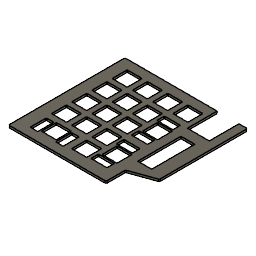
numpad (Autodesk Fusion 360 archive; units mm, degrees)
design "middle"
part number: 2026-06-12-14-33-51-478
Autodesk Fusion 360 part; units mm, degrees
sketch "Sketch2" plane through (0, 0, 0) normal (0, 0, 1) x (1, 0, 0)
  line L0 (-33.9143, 32.5199) -> (-20.9143, 32.5199)
  line L1 (-33.9143, 18.5199) -> (-20.9143, 18.5199)
  line L2 (-34.4143, 32.0199) -> (-34.4143, 19.0199)
  line L3 (-20.4143, 32.0199) -> (-20.4143, 19.0199)
  arc A0 (-33.9143, 32.5199) -> (-34.4143, 32.0199) centre (-33.9143, 32.0199) ccw
  arc A1 (-20.4143, 32.0199) -> (-20.9143, 32.5199) centre (-20.9143, 32.0199) ccw
  arc A2 (-34.4143, 19.0199) -> (-33.9143, 18.5199) centre (-33.9143, 19.0199) ccw
  arc A3 (-20.9143, 18.5199) -> (-20.4143, 19.0199) centre (-20.9143, 19.0199) ccw
  line L4 (-14.8643, 32.5199) -> (-1.8643, 32.5199)
  line L5 (-14.8643, 18.5199) -> (-1.8643, 18.5199)
  line L6 (-15.3643, 32.0199) -> (-15.3643, 19.0199)
  line L7 (-1.3643, 32.0199) -> (-1.3643, 19.0199)
  arc A4 (-14.8643, 32.5199) -> (-15.3643, 32.0199) centre (-14.8643, 32.0199) ccw
  arc A5 (-1.3643, 32.0199) -> (-1.8643, 32.5199) centre (-1.8643, 32.0199) ccw
  arc A6 (-15.3643, 19.0199) -> (-14.8643, 18.5199) centre (-14.8643, 19.0199) ccw
  arc A7 (-1.8643, 18.5199) -> (-1.3643, 19.0199) centre (-1.8643, 19.0199) ccw
  line L8 (4.1857, 32.5199) -> (17.1857, 32.5199)
  line L9 (4.1857, 18.5199) -> (17.1857, 18.5199)
  line L10 (3.6857, 32.0199) -> (3.6857, 19.0199)
  line L11 (17.6857, 32.0199) -> (17.6857, 19.0199)
  arc A8 (4.1857, 32.5199) -> (3.6857, 32.0199) centre (4.1857, 32.0199) ccw
  arc A9 (17.6857, 32.0199) -> (17.1857, 32.5199) centre (17.1857, 32.0199) ccw
  arc A10 (3.6857, 19.0199) -> (4.1857, 18.5199) centre (4.1857, 19.0199) ccw
  arc A11 (17.1857, 18.5199) -> (17.6857, 19.0199) centre (17.1857, 19.0199) ccw
  line L12 (23.2357, 32.5199) -> (36.2357, 32.5199)
  line L13 (23.2357, 18.5199) -> (36.2357, 18.5199)
  line L14 (22.7357, 32.0199) -> (22.7357, 19.0199)
  line L15 (36.7357, 32.0199) -> (36.7357, 19.0199)
  arc A12 (23.2357, 32.5199) -> (22.7357, 32.0199) centre (23.2357, 32.0199) ccw
  arc A13 (36.7357, 32.0199) -> (36.2357, 32.5199) centre (36.2357, 32.0199) ccw
  arc A14 (22.7357, 19.0199) -> (23.2357, 18.5199) centre (23.2357, 19.0199) ccw
  arc A15 (36.2357, 18.5199) -> (36.7357, 19.0199) centre (36.2357, 19.0199) ccw
  line L16 (-33.9143, 13.4699) -> (-20.9143, 13.4699)
  line L17 (-33.9143, -0.5301) -> (-20.9143, -0.5301)
  line L18 (-34.4143, 12.9699) -> (-34.4143, -0.0301)
  line L19 (-20.4143, 12.9699) -> (-20.4143, -0.0301)
  arc A16 (-33.9143, 13.4699) -> (-34.4143, 12.9699) centre (-33.9143, 12.9699) ccw
  arc A17 (-20.4143, 12.9699) -> (-20.9143, 13.4699) centre (-20.9143, 12.9699) ccw
  arc A18 (-34.4143, -0.0301) -> (-33.9143, -0.5301) centre (-33.9143, -0.0301) ccw
  arc A19 (-20.9143, -0.5301) -> (-20.4143, -0.0301) centre (-20.9143, -0.0301) ccw
  line L20 (-14.8643, 13.4699) -> (-1.8643, 13.4699)
  line L21 (-14.8643, -0.5301) -> (-1.8643, -0.5301)
  line L22 (-15.3643, 12.9699) -> (-15.3643, -0.0301)
  line L23 (-1.3643, 12.9699) -> (-1.3643, -0.0301)
  arc A20 (-14.8643, 13.4699) -> (-15.3643, 12.9699) centre (-14.8643, 12.9699) ccw
  arc A21 (-1.3643, 12.9699) -> (-1.8643, 13.4699) centre (-1.8643, 12.9699) ccw
  arc A22 (-15.3643, -0.0301) -> (-14.8643, -0.5301) centre (-14.8643, -0.0301) ccw
  arc A23 (-1.8643, -0.5301) -> (-1.3643, -0.0301) centre (-1.8643, -0.0301) ccw
  line L24 (4.1857, 13.4699) -> (17.1857, 13.4699)
  line L25 (4.1857, -0.5301) -> (17.1857, -0.5301)
  line L26 (3.6857, 12.9699) -> (3.6857, -0.0301)
  line L27 (17.6857, 12.9699) -> (17.6857, -0.0301)
  arc A24 (4.1857, 13.4699) -> (3.6857, 12.9699) centre (4.1857, 12.9699) ccw
  arc A25 (17.6857, 12.9699) -> (17.1857, 13.4699) centre (17.1857, 12.9699) ccw
  arc A26 (3.6857, -0.0301) -> (4.1857, -0.5301) centre (4.1857, -0.0301) ccw
  arc A27 (17.1857, -0.5301) -> (17.6857, -0.0301) centre (17.1857, -0.0301) ccw
  line L28 (36.7357, 3.4449) -> (36.7357, -9.5551)
  line L29 (22.7357, 3.4449) -> (22.7357, -9.5551)
  line L30 (36.2357, 3.9449) -> (23.2357, 3.9449)
  line L31 (36.2357, -10.0551) -> (23.2357, -10.0551)
  arc A28 (36.7357, 3.4449) -> (36.2357, 3.9449) centre (36.2357, 3.4449) ccw
  arc A29 (36.2357, -10.0551) -> (36.7357, -9.5551) centre (36.2357, -9.5551) ccw
  arc A30 (23.2357, 3.9449) -> (22.7357, 3.4449) centre (23.2357, 3.4449) ccw
  arc A31 (22.7357, -9.5551) -> (23.2357, -10.0551) centre (23.2357, -9.5551) ccw
  line L32 (35.7357, 11.8829) -> (35.7357, 5.8829)
  line L33 (20.7357, 11.8829) -> (20.7357, 5.8829)
  line L34 (35.2357, 12.3829) -> (21.2357, 12.3829)
  line L35 (35.2357, 5.3829) -> (21.2357, 5.3829)
  arc A32 (35.7357, 11.8829) -> (35.2357, 12.3829) centre (35.2357, 11.8829) ccw
  arc A33 (35.2357, 5.3829) -> (35.7357, 5.8829) centre (35.2357, 5.8829) ccw
  arc A34 (21.2357, 12.3829) -> (20.7357, 11.8829) centre (21.2357, 11.8829) ccw
  arc A35 (20.7357, 5.8829) -> (21.2357, 5.3829) centre (21.2357, 5.8829) ccw
  line L36 (35.7357, -11.9931) -> (35.7357, -17.9931)
  line L37 (20.7357, -11.9931) -> (20.7357, -17.9931)
  line L38 (35.2357, -11.4931) -> (21.2357, -11.4931)
  line L39 (35.2357, -18.4931) -> (21.2357, -18.4931)
  arc A36 (35.7357, -11.9931) -> (35.2357, -11.4931) centre (35.2357, -11.9931) ccw
  arc A37 (35.2357, -18.4931) -> (35.7357, -17.9931) centre (35.2357, -17.9931) ccw
  arc A38 (21.2357, -11.4931) -> (20.7357, -11.9931) centre (21.2357, -11.9931) ccw
  arc A39 (20.7357, -17.9931) -> (21.2357, -18.4931) centre (21.2357, -17.9931) ccw
  line L40 (-33.9143, -5.5801) -> (-20.9143, -5.5801)
  line L41 (-33.9143, -19.5801) -> (-20.9143, -19.5801)
  line L42 (-34.4143, -6.0801) -> (-34.4143, -19.0801)
  line L43 (-20.4143, -6.0801) -> (-20.4143, -19.0801)
  arc A40 (-33.9143, -5.5801) -> (-34.4143, -6.0801) centre (-33.9143, -6.0801) ccw
  arc A41 (-20.4143, -6.0801) -> (-20.9143, -5.5801) centre (-20.9143, -6.0801) ccw
  arc A42 (-34.4143, -19.0801) -> (-33.9143, -19.5801) centre (-33.9143, -19.0801) ccw
  arc A43 (-20.9143, -19.5801) -> (-20.4143, -19.0801) centre (-20.9143, -19.0801) ccw
  line L44 (-14.8643, -5.5801) -> (-1.8643, -5.5801)
  line L45 (-14.8643, -19.5801) -> (-1.8643, -19.5801)
  line L46 (-15.3643, -6.0801) -> (-15.3643, -19.0801)
  line L47 (-1.3643, -6.0801) -> (-1.3643, -19.0801)
  arc A44 (-14.8643, -5.5801) -> (-15.3643, -6.0801) centre (-14.8643, -6.0801) ccw
  arc A45 (-1.3643, -6.0801) -> (-1.8643, -5.5801) centre (-1.8643, -6.0801) ccw
  arc A46 (-15.3643, -19.0801) -> (-14.8643, -19.5801) centre (-14.8643, -19.0801) ccw
  arc A47 (-1.8643, -19.5801) -> (-1.3643, -19.0801) centre (-1.8643, -19.0801) ccw
  line L48 (4.1857, -5.5801) -> (17.1857, -5.5801)
  line L49 (4.1857, -19.5801) -> (17.1857, -19.5801)
  line L50 (3.6857, -6.0801) -> (3.6857, -19.0801)
  line L51 (17.6857, -6.0801) -> (17.6857, -19.0801)
  arc A48 (4.1857, -5.5801) -> (3.6857, -6.0801) centre (4.1857, -6.0801) ccw
  arc A49 (17.6857, -6.0801) -> (17.1857, -5.5801) centre (17.1857, -6.0801) ccw
  arc A50 (3.6857, -19.0801) -> (4.1857, -19.5801) centre (4.1857, -19.0801) ccw
  arc A51 (17.1857, -19.5801) -> (17.6857, -19.0801) centre (17.1857, -19.0801) ccw
  line L52 (-33.9143, -24.6301) -> (-20.9143, -24.6301)
  line L53 (-33.9143, -38.6301) -> (-20.9143, -38.6301)
  line L54 (-34.4143, -25.1301) -> (-34.4143, -38.1301)
  line L55 (-20.4143, -25.1301) -> (-20.4143, -38.1301)
  arc A52 (-33.9143, -24.6301) -> (-34.4143, -25.1301) centre (-33.9143, -25.1301) ccw
  arc A53 (-20.4143, -25.1301) -> (-20.9143, -24.6301) centre (-20.9143, -25.1301) ccw
  arc A54 (-34.4143, -38.1301) -> (-33.9143, -38.6301) centre (-33.9143, -38.1301) ccw
  arc A55 (-20.9143, -38.6301) -> (-20.4143, -38.1301) centre (-20.9143, -38.1301) ccw
  line L56 (-14.8643, -24.6301) -> (-1.8643, -24.6301)
  line L57 (-14.8643, -38.6301) -> (-1.8643, -38.6301)
  line L58 (-15.3643, -25.1301) -> (-15.3643, -38.1301)
  line L59 (-1.3643, -25.1301) -> (-1.3643, -38.1301)
  arc A56 (-14.8643, -24.6301) -> (-15.3643, -25.1301) centre (-14.8643, -25.1301) ccw
  arc A57 (-1.3643, -25.1301) -> (-1.8643, -24.6301) centre (-1.8643, -25.1301) ccw
  arc A58 (-15.3643, -38.1301) -> (-14.8643, -38.6301) centre (-14.8643, -38.1301) ccw
  arc A59 (-1.8643, -38.6301) -> (-1.3643, -38.1301) centre (-1.8643, -38.1301) ccw
  line L60 (4.1857, -24.6301) -> (17.1857, -24.6301)
  line L61 (4.1857, -38.6301) -> (17.1857, -38.6301)
  line L62 (3.6857, -25.1301) -> (3.6857, -38.1301)
  line L63 (17.6857, -25.1301) -> (17.6857, -38.1301)
  arc A60 (4.1857, -24.6301) -> (3.6857, -25.1301) centre (4.1857, -25.1301) ccw
  arc A61 (17.6857, -25.1301) -> (17.1857, -24.6301) centre (17.1857, -25.1301) ccw
  arc A62 (3.6857, -38.1301) -> (4.1857, -38.6301) centre (4.1857, -38.1301) ccw
  arc A63 (17.1857, -38.6301) -> (17.6857, -38.1301) centre (17.1857, -38.1301) ccw
  line L64 (36.7357, -34.6551) -> (36.7357, -47.6551)
  line L65 (22.7357, -34.6551) -> (22.7357, -47.6551)
  line L66 (36.2357, -34.1551) -> (23.2357, -34.1551)
  line L67 (36.2357, -48.1551) -> (23.2357, -48.1551)
  arc A64 (36.7357, -34.6551) -> (36.2357, -34.1551) centre (36.2357, -34.6551) ccw
  arc A65 (36.2357, -48.1551) -> (36.7357, -47.6551) centre (36.2357, -47.6551) ccw
  arc A66 (23.2357, -34.1551) -> (22.7357, -34.6551) centre (23.2357, -34.6551) ccw
  arc A67 (22.7357, -47.6551) -> (23.2357, -48.1551) centre (23.2357, -47.6551) ccw
  line L68 (35.7357, -26.2171) -> (35.7357, -32.2171)
  line L69 (20.7357, -26.2171) -> (20.7357, -32.2171)
  line L70 (35.2357, -25.7171) -> (21.2357, -25.7171)
  line L71 (35.2357, -32.7171) -> (21.2357, -32.7171)
  arc A68 (35.7357, -26.2171) -> (35.2357, -25.7171) centre (35.2357, -26.2171) ccw
  arc A69 (35.2357, -32.7171) -> (35.7357, -32.2171) centre (35.2357, -32.2171) ccw
  arc A70 (21.2357, -25.7171) -> (20.7357, -26.2171) centre (21.2357, -26.2171) ccw
  arc A71 (20.7357, -32.2171) -> (21.2357, -32.7171) centre (21.2357, -32.2171) ccw
  line L72 (35.7357, -50.0931) -> (35.7357, -56.0931)
  line L73 (20.7357, -50.0931) -> (20.7357, -56.0931)
  line L74 (35.2357, -49.5931) -> (21.2357, -49.5931)
  line L75 (35.2357, -56.5931) -> (21.2357, -56.5931)
  arc A72 (35.7357, -50.0931) -> (35.2357, -49.5931) centre (35.2357, -50.0931) ccw
  arc A73 (35.2357, -56.5931) -> (35.7357, -56.0931) centre (35.2357, -56.0931) ccw
  arc A74 (21.2357, -49.5931) -> (20.7357, -50.0931) centre (21.2357, -50.0931) ccw
  arc A75 (20.7357, -56.0931) -> (21.2357, -56.5931) centre (21.2357, -56.0931) ccw
  line L76 (-24.3893, -43.6801) -> (-11.3893, -43.6801)
  line L77 (-24.3893, -57.6801) -> (-11.3893, -57.6801)
  line L78 (-24.8893, -44.1801) -> (-24.8893, -57.1801)
  line L79 (-10.8893, -44.1801) -> (-10.8893, -57.1801)
  arc A76 (-24.3893, -43.6801) -> (-24.8893, -44.1801) centre (-24.3893, -44.1801) ccw
  arc A77 (-10.8893, -44.1801) -> (-11.3893, -43.6801) centre (-11.3893, -44.1801) ccw
  arc A78 (-24.8893, -57.1801) -> (-24.3893, -57.6801) centre (-24.3893, -57.1801) ccw
  arc A79 (-11.3893, -57.6801) -> (-10.8893, -57.1801) centre (-11.3893, -57.1801) ccw
  line L80 (-32.8273, -44.6801) -> (-26.8273, -44.6801)
  line L81 (-32.8273, -59.6801) -> (-26.8273, -59.6801)
  line L82 (-33.3273, -45.1801) -> (-33.3273, -59.1801)
  line L83 (-26.3273, -45.1801) -> (-26.3273, -59.1801)
  arc A80 (-32.8273, -44.6801) -> (-33.3273, -45.1801) centre (-32.8273, -45.1801) ccw
  arc A81 (-26.3273, -45.1801) -> (-26.8273, -44.6801) centre (-26.8273, -45.1801) ccw
  arc A82 (-33.3273, -59.1801) -> (-32.8273, -59.6801) centre (-32.8273, -59.1801) ccw
  arc A83 (-26.8273, -59.6801) -> (-26.3273, -59.1801) centre (-26.8273, -59.1801) ccw
  line L84 (-8.9513, -44.6801) -> (-2.9513, -44.6801)
  line L85 (-8.9513, -59.6801) -> (-2.9513, -59.6801)
  line L86 (-9.4513, -45.1801) -> (-9.4513, -59.1801)
  line L87 (-2.4513, -45.1801) -> (-2.4513, -59.1801)
  arc A84 (-8.9513, -44.6801) -> (-9.4513, -45.1801) centre (-8.9513, -45.1801) ccw
  arc A85 (-2.4513, -45.1801) -> (-2.9513, -44.6801) centre (-2.9513, -45.1801) ccw
  arc A86 (-9.4513, -59.1801) -> (-8.9513, -59.6801) centre (-8.9513, -59.1801) ccw
  arc A87 (-2.9513, -59.6801) -> (-2.4513, -59.1801) centre (-2.9513, -59.1801) ccw
  line L88 (4.1857, -43.6801) -> (17.1857, -43.6801)
  line L89 (4.1857, -57.6801) -> (17.1857, -57.6801)
  line L90 (3.6857, -44.1801) -> (3.6857, -57.1801)
  line L91 (17.6857, -44.1801) -> (17.6857, -57.1801)
  arc A88 (4.1857, -43.6801) -> (3.6857, -44.1801) centre (4.1857, -44.1801) ccw
  arc A89 (17.6857, -44.1801) -> (17.1857, -43.6801) centre (17.1857, -44.1801) ccw
  arc A90 (3.6857, -57.1801) -> (4.1857, -57.6801) centre (4.1857, -57.1801) ccw
  arc A91 (17.1857, -57.6801) -> (17.6857, -57.1801) centre (17.1857, -57.1801) ccw
  line L92 (-45.3643, 41.3839) -> (-45.3643, -68.2151)
  line L93 (-40.3643, -63.2151) -> (-40.3643, 36.3843)
  line L94 (-40.3643, 36.3843) -> (63.6858, 36.3349)
  line L95 (63.6858, -36.4651) -> (41.4358, -44.9151)
  line L96 (63.6858, 36.3349) -> (63.6858, -36.4651)
  line L97 (41.4358, -63.2151) -> (-40.3643, -63.2151)
  line L98 (41.4358, -44.9151) -> (41.4358, -63.2151)
  line L99 (69.9584, -41.4651) -> (69.9584, 41.3349)
  line L100 (-45.3643, -68.2151) -> (46.4357, -68.2151)
  line L101 (46.4357, -49.9317) -> (69.9584, -41.4651)
  line L102 (69.9584, 41.3349) -> (-45.3643, 41.3839)
  line L103 (46.4357, -68.2151) -> (46.4357, -49.9317)
  line L104 (41.5, 41.347) -> (62, 41.347)
  line L105 (62, 41.347) -> (62, 13.3572)
  line L106 (62, 13.3572) -> (41.5, 13.3572)
  line L107 (41.5, 13.3572) -> (41.5, 41.347)
  line L108 (44.9584, 3.6646) -> (57.9584, 3.6646)
  line L109 (57.9584, 3.6646) -> (57.9584, -36.8091)
  line L110 (57.9584, -36.8091) -> (44.9584, -36.8091)
  line L111 (44.9584, -36.8091) -> (44.9584, 3.6646)
  dimension "d1" = 5
  dimension "d2" = 109.599
  dimension "d3" = 91.8
  dimension "d4" = 5
  dimension "d5" = 5
  dimension "d6" = 25
  dimension "d7" = 1
  dimension "d8" = 5
  dimension "d9" = 10.535
  dimension "d10" = 20.475
  dimension "d11" = 20.5
  dimension "d12" = 13
  dimension "d14" = 12
  constraint vertical L96
  constraint parallel L96 L98
  constraint perpendicular L97 L98
  constraint parallel L92 L93
  constraint perpendicular L92 L100
  constraint perpendicular L100 L103
  constraint vertical L99
  constraint horizontal L104
  constraint vertical L105
  constraint horizontal L106
  constraint vertical L107
  constraint coincident L102 L104.start
  constraint horizontal L108
  constraint vertical L109
  constraint horizontal L110
  constraint vertical L111
  measures "d1" distance of L92 L93
  measures "d2" vertical distance of L92.start L92.end
  measures "d3" horizontal distance of L92.end L100.end
  measures "d4" distance of L97 L100
  measures "d5" vertical distance of L95.start L99.start
  measures "d6" distance of L99.start L101.start
  measures "d7" angle of L95 L101
  measures "d8" vertical distance of L99.end L94.end
  measures "d9" distance of L77 L100
  measures "d10" distance of L78 L92
  measures "d11" distance of L105 L107
  measures "d12" distance of L109 L111
  measures "d14" distance of L99 L109
extrude "Extrude1" add sketch "Sketch2" along normal blind 2 contours L92 L93 L94 L95 L96 L97 L98 L99 L100 L101 L102 L103 L105 L107 | L93 L94 L95 L96 L97 L98 L105 L106 L107
fillet "Fillet1" radius 1 6 edges at (-45.3643, -68.2151, 1) (-45.3643, 41.3839, 1) (69.9584, 41.3349, 1) (69.9584, -41.4651, 1) (46.4357, -49.9317, 1) (46.4357, -68.2151, 1)
